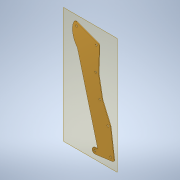
# Autodesk Inventor part: side skert v2
Saved by Autodesk Inventor 2020 (Build 240168000, 168)
## iProperties
Created: 2022-08-10
Part Number: side skert v2
Material: Brass, Soft Yellow
Document SubType Name: Modeling
Designer: Steven
Density: 8.47 g/cm^3
Appearance: Brass - Satin
Mass: 43.6224 g
Surface Area: 107.877 cm^2
Volume: 5.15022 cm^3
Author: Steven
Autodesk Inventor part; units mm, degrees
ref_plane "YZ Plane" through (0, 0, 0) normal (1, 0, 0) x (0, 1, 0)
ref_plane "XZ Plane" through (0, 0, 0) normal (0, 1, 0) x (-1, 0, 0)
ref_plane "XY Plane" through (0, 0, 0) normal (0, 0, 1) x (1, 0, 0)
ref_plane "Work Plane1" through (0, 0, 0) normal (0, 0, 1) x (1, 0, 0)
sketch "Sketch1" plane through (0, 0, 0) normal (0, 0, 1) x (1, 0, 0)
  line L0 (12.6235, -7.6637) -> (25.0692, -36.6156) projected
  arc A0 (25.2873, -37.408) -> (25.0692, -36.6156) centre (22.3131, -37.8003) ccw projected
  line L1 (25.2873, -37.408) -> (29.8752, -72.1865) projected
  arc A1 (28.1539, -74.4309) -> (29.8752, -72.1865) centre (27.8924, -72.448) ccw projected
  line L2 (28.1539, -74.4309) -> (7.7764, -77.119) projected
  arc A2 (7.7764, -77.119) -> (8.9535, -86.0417) centre (8.365, -81.5803) ccw projected
  line L3 (8.9535, -86.0417) -> (37.2623, -82.3073) projected
  arc A3 (37.2623, -82.3073) -> (39.8442, -78.9407) centre (36.8699, -79.3331) ccw projected
  line L4 (39.8442, -78.9407) -> (34.0473, -34.997) projected
  arc A4 (34.0473, -34.997) -> (33.8292, -34.2046) centre (31.073, -35.3894) ccw projected
  line L5 (33.8292, -34.2046) -> (20.8924, -4.1103) projected
  arc A5 (20.4398, -2.6174) -> (20.8924, -4.1103) centre (27.3234, -1.3458) ccw projected
  line L6 (20.4398, -2.6174) -> (14.5173, 29.4432) projected
  arc A6 (14.405, 30.9564) -> (14.5173, 29.4432) centre (21.4008, 30.7148) ccw projected
  line L7 (14.405, 30.9564) -> (15.7585, 70.1518) projected
  arc A7 (15.7585, 70.1518) -> (13.7755, 73.0784) centre (12.7603, 70.2554) ccw projected
  line L8 (13.7755, 73.0784) -> (-21.8863, 85.9033) projected
  arc A8 (-21.8863, 85.9033) -> (-25.7246, 84.0956) centre (-22.9016, 83.0803) ccw projected
  line L9 (-25.7246, 84.0956) -> (-39.6044, 45.5005) projected
  arc A9 (-39.6044, 45.5005) -> (-31.1354, 42.4548) centre (-35.3699, 43.9777) ccw projected
  line L10 (-31.1354, 42.4548) -> (-28.9682, 48.481) projected
  arc A10 (-23.2109, 51.1927) -> (-28.9682, 48.481) centre (-24.7337, 46.9582) ccw projected
  line L11 (-23.2109, 51.1927) -> (2.9943, 41.7686) projected
  arc A11 (5.6382, 37.8666) -> (2.9943, 41.7686) centre (1.6406, 38.0046) ccw projected
  line L12 (5.6382, 37.8666) -> (5.4104, 31.2681) projected
  arc A12 (5.4104, 31.2681) -> (5.5231, 29.7528) centre (12.4062, 31.0266) ccw projected
  line L13 (5.5231, 29.7528) -> (12.1714, -6.1729) projected
  arc A13 (12.1714, -6.1729) -> (12.6235, -7.6637) centre (19.0545, -4.8992) ccw projected
  circle A14 centre (29.5855, -35.7988) radius 1.55 projected
  circle A15 centre (10.5349, 68.7475) radius 1.55 projected
  circle A16 centre (16.4901, -5.1537) radius 1.55 projected
  circle A17 centre (-21.4682, 80.037) radius 1.55 projected
  circle A18 centre (-35.3699, 43.9777) radius 1.55 projected
  circle A19 centre (34.3649, -77.4119) radius 1.55 projected
  circle A20 centre (-28.5644, 59.2229) radius 1.55 projected
  circle A21 centre (8.365, -81.5803) radius 1.55 projected
  circle A22 centre (9.9227, 30.3521) radius 1.55 projected
  line L14 (0.9032, 52.0849) -> (-20.6357, 59.8309) projected
  arc A23 (-23.0461, 64.9485) -> (-20.6357, 59.8309) centre (-19.2821, 63.5949) ccw projected
  line L15 (-23.0461, 64.9485) -> (-20.3013, 72.5809) projected
  arc A24 (-16.463, 74.3887) -> (-20.3013, 72.5809) centre (-17.4783, 71.5657) ccw projected
  line L16 (-16.463, 74.3887) -> (3.8682, 67.077) projected
  arc A25 (6.5122, 63.1749) -> (3.8682, 67.077) centre (2.5146, 63.313) ccw projected
  line L17 (6.5122, 63.1749) -> (6.2544, 55.7109) projected
  arc A26 (0.9032, 52.0849) -> (6.2544, 55.7109) centre (2.2568, 55.8489) ccw projected
  line L18 (-14.3316, 28.4241) -> (-19.7537, 49.0626) construction
  line L19 (1.5801, -32.1414) -> (-3.5777, -12.5091) construction
  line L20 (-6.8942, 0.1146) -> (-11.0151, 15.8005) construction
  line L21 (-25.7315, 60.0097) -> (-31.5346, 58.4851) construction
  line L22 (-19.8838, 37.7512) -> (-25.7315, 60.0097) construction
  line L23 (-25.6869, 36.2266) -> (-19.8838, 37.7512) construction
  line L24 (-25.6869, 36.2266) -> (-31.5346, 58.4851) construction
  line L25 (1.5128, -67.305) -> (7.3158, -65.7804) construction
  line L26 (10.8632, -102.8959) -> (1.5128, -67.305) construction
  line L27 (16.6662, -101.3713) -> (10.8632, -102.8959) construction
  line L28 (7.3158, -65.7804) -> (16.6662, -101.3713) construction
  line L29 (-20.011, 50.0419) -> (13.2082, -76.4024)
  arc A27 (-27.5927, 78.9008) -> (-20.011, 50.0419) centre (8.9141, 73.0664) ccw
  point P0 (0, 0)
  constraints: 4 point on line, 2 end point, 2 point on circle, 1 centre point, 1 parallel
extrude "Extrusion1" add sketch "Sketch1" along normal blind 1 contours A13 L13 A12 L12 A11 L11 A27 L9 A8 L8 A7 L7 A6 L6 A5 L5 A4 L4 A3 L3 A2 L2 A1 L1 A0 L0 | L0 A0 L1 A1 L2 L29 L11 A11 L12 A12 L13 A13 | L14 A23 L15 A24 L16 A25 L17 A26
body "Solid1"
